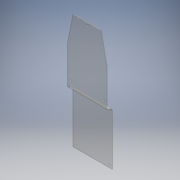
# Autodesk Inventor part: cover
Saved by Autodesk Inventor 2016 (Build 200138000, 138)
## iProperties
Created: 2016-09-23
Part Number: cover
Material: PET Plastic
Document SubType Name: Modeling
Designer: Jakub
Density: 1.541 g/cm^3
Appearance: Polycarbonate - Clear
Author: Jakub
Autodesk Inventor part; units mm, degrees
ref_plane "YZ Plane" through (0, 0, 0) normal (1, 0, 0) x (0, 1, 0)
ref_plane "XZ Plane" through (0, 0, 0) normal (0, 1, 0) x (-1, 0, 0)
ref_plane "XY Plane" through (0, 0, 0) normal (0, 0, 1) x (1, 0, 0)
sketch "Sketch1" plane through (0, 0, 0) normal (1, 0, 0) x (0, 1, 0)
  line L0 (-0.5, 45) -> (0.5, 45)
  line L1 (0.5, 45) -> (0.5, -45)
  line L2 (0.5, -45) -> (-0.5, -45)
  line L3 (-0.5, -45) -> (-0.5, 45)
  line L4 (-0.5, 45) -> (0.5, -45) construction
  line L5 (0.5, 45) -> (-0.5, -45) construction
  line L6 (-0.5, 45) -> (-5.5, 45)
  line L7 (-5.5, 45) -> (-5.5, 50)
  line L8 (-5.5, 50) -> (-10.5, 50)
  line L9 (-10.5, 50) -> (-10.5, 55)
  arc A0 (-0.5, 45) -> (-5.5, 50) centre (-5.5, 45) ccw
  arc A1 (-10.5, 55) -> (-5.5, 50) centre (-5.5, 55) ccw
  line L10 (-5.5, 50) -> (-5.5, 51)
  arc A2 (0.5, 45) -> (-5.5, 51) centre (-5.5, 45) ccw
  line L11 (-10.5, 55) -> (-9.5, 55)
  line L12 (-10.5, 55) -> (-9.5, 55)
  line L13 (-9.5, 55) -> (-9.5, 165)
  line L14 (-9.5, 165) -> (-10.5, 165)
  line L15 (-10.5, 165) -> (-10.5, 55)
  arc A3 (-9.5, 55) -> (-5.5, 51) centre (-5.5, 55) ccw
  point P0 (0, 0)
  dimension "d0" = 1
  dimension "d1" = 90
  dimension "d2" = 5
  dimension "d3" = 5
  dimension "d4" = 5
  dimension "d5" = 5
  dimension "d6" = 5
  dimension "d7" = 5
  dimension "d8" = 1
  dimension "d9" = 6
  dimension "d10" = 1
  dimension "d12" = 1
  dimension "d13" = 110
  dimension "d14" = 4
  constraints: 32 end point, 8 point on circle, 5 perpendicular, 4 centre point, 4 horizontal, 4 parallel, 2 midpoint, 1 vertical
  measures "d0" distance of L1.end L2.end
  measures "d1" distance of L0.end L1.end
  measures "d2" distance of L0.start L6.end
  measures "d3" distance of L6.end L7.end
  measures "d4" distance of L7.end L8.end
  measures "d5" distance of L8.end L9.end
  measures "d6" radius of A0
  measures "d7" radius of A1
  measures "d8" distance of L7.end L10.end
  measures "d9" radius of A2
  measures "d10" distance of L9.end L11.end
  measures "d12" distance of L14.end L13.end
  measures "d13" distance of L13.end L12.end
  measures "d14" radius of A3
extrude "Extrusion1" add sketch "Sketch1" along normal blind 70 contours A0 L10 A2 L0 | L0 L1 L2 L3 | A1 L11 A3 L10 | L15 L14 L13 L11
sketch "Sketch2" plane through (0, 0.5, 45) normal (0, 1, 0) x (1, 0, 0)
  circle A0 centre (5, 85) radius 1.5
  circle A1 centre (65, 85) radius 1.5
  line L0 (0, 90) -> (70, 90) projected
  line L1 (70, 90) -> (70, 0) projected
  line L2 (0, 90) -> (0, 0) projected
  point P0 (0, 45)
  dimension "d17" = 3
  dimension "d18" = 3
  dimension "d19" = 5
  dimension "d20" = 5
  dimension "d21" = 5
  dimension "d22" = 5
  constraints: 2 centre point
  measures "d17" diameter of A0
  measures "d18" diameter of A1
  measures "d19" distance from line of L0 A1.centre
  measures "d20" distance from line of L1 A1.centre
  measures "d21" distance from line of L0 A0.centre
  measures "d22" distance from line of L2 A0.centre
extrude "Extrusion2" cut sketch "Sketch2" against normal up to next
sketch "Sketch3" plane through (0, -9.5, 165) normal (0, 1, 0) x (1, 0, 0)
  circle A0 centre (5, 100) radius 1.5
  circle A1 centre (65, 100) radius 1.5
  line L0 (0, 110) -> (70, 110) projected
  line L1 (70, 110) -> (70, 0) projected
  line L2 (0, 110) -> (0, 0) projected
  point P0 (0, 165)
  dimension "d25" = 3
  dimension "d26" = 3
  dimension "d27" = 10
  dimension "d28" = 5
  dimension "d29" = 10
  dimension "d30" = 5
  constraints: 2 centre point
  measures "d25" diameter of A0
  measures "d26" diameter of A1
  measures "d27" distance from line of L0 A1.centre
  measures "d28" distance from line of L1 A1.centre
  measures "d29" distance from line of L0 A0.centre
  measures "d30" distance from line of L2 A0.centre
extrude "Extrusion3" cut sketch "Sketch3" against normal up to next
sketch "Sketch4" plane through (0, -10.5, 165) normal (0, 0, 1) x (1, 0, 0)
  line L0 (0, 0) -> (70, 0) projected
  line L1 (0, 0) -> (70, 0)
  line L2 (70, 0) -> (70, 1)
  line L3 (70, 1) -> (0, 1)
  line L4 (0, 1) -> (0, 0)
  point P0 (0, 10.5)
  constraints: 8 end point, 2 parallel, 1 horizontal, 1 perpendicular
extrude "Extrusion4" add sketch "Sketch4" along normal blind 5.5
sketch "Sketch5" plane through (0, -9.5, 55) normal (0, 1, 0) x (1, 0, 0)
  line L0 (70, -115.5) -> (0, -115.5) projected
  line L1 (35, -115.5) -> (35, -110.5)
  circle A0 centre (35, -110.5) radius 1.5
  point P0 (0, 55)
  dimension "d35" = 5
  dimension "d36" = 3
  constraints: 2 end point, 1 centre point, 1 coincident, 1 midpoint, 1 vertical
  measures "d35" distance of L1.start L1.end
  measures "d36" diameter of A0
extrude "Extrusion5" cut sketch "Sketch5" against normal up to next
sketch "Sketch6" plane through (0, -9.5, 55) normal (0, 1, 0) x (1, 0, 0)
  line L0 (70, -115.5) -> (0, -115.5) projected
  line L1 (35, -115.5) -> (60, -115.5)
  line L2 (35, -115.5) -> (10, -115.5)
  line L3 (0, -115.5) -> (0, -65.5)
  line L4 (0, 0) -> (0, -115.5) projected
  line L5 (70, -115.5) -> (70, -65.5)
  line L6 (70, 0) -> (70, -115.5) projected
  line L7 (70, -65.5) -> (60, -115.5)
  line L8 (0, -65.5) -> (10, -115.5)
  line L9 (10, -115.5) -> (0, -115.5)
  line L10 (60, -115.5) -> (70, -115.5)
  point P0 (0, 55)
  dimension "d39" = 25
  dimension "d40" = 25
  dimension "d41" = 50
  dimension "d42" = 50
  constraints: 16 end point, 4 point on line, 1 collinear, 1 midpoint, 1 perpendicular
  measures "d39" distance of L1.start L1.end
  measures "d40" distance of L1.start L2.end
  measures "d41" distance of L0.end L3.end
  measures "d42" distance of L0.start L5.end
extrude "Extrusion6" cut sketch "Sketch6" against normal up to next
body "Solid1"
